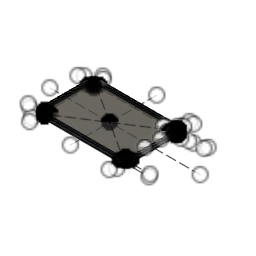
cover_bottom v1 (Autodesk Fusion 360 design; units mm, degrees)
Autodesk Fusion 360 part; units mm, degrees
note: some values were not read from the file. Set by a fixed rule: the direction of a hole.
sketch "Skizze1" plane through (0, 0, 0) normal (0, 0, 1) x (1, 0, 0)
  line L0 (85, -55) -> (-85, -55) construction
  line L1 (-85, -55) -> (-85, 55) construction
  line L2 (-85, 55) -> (85, 55) construction
  line L3 (85, 55) -> (85, -55) construction
  line L4 (85, -55) -> (-85, 55) construction
  line L5 (-85, -55) -> (85, 55) construction
  line L6 (83.8, -53.8) -> (-83.8, -53.8) construction
  line L7 (-83.8, -53.8) -> (-83.8, 53.8) construction
  line L8 (-83.8, 53.8) -> (83.8, 53.8) construction
  line L9 (83.8, 53.8) -> (83.8, -53.8) construction
  line L10 (83.8, -53.8) -> (-83.8, 53.8) construction
  line L11 (-83.8, -53.8) -> (83.8, 53.8) construction
  line L12 (60, 45) -> (112.6344, 45) construction
  line L13 (75, 65.4743) -> (75, 20.9271) construction
  arc A0 (85, 45) -> (75, 55) centre (75, 45) ccw
  line L14 (74, 76.2401) -> (74, -7.7296) construction
  line L15 (56.5373, 44) -> (104.4576, 44) construction
  arc A1 (83.8, 44) -> (74, 53.8) centre (74, 44) ccw
  line L16 (69, 40.8) -> (92.7084, 40.8) construction
  line L17 (70.8, 58.1175) -> (70.8, 37.2449) construction
  line L18 (-99.6173, 51.6) -> (133.2089, 51.6) construction
  line L19 (-98.318, -51.6) -> (125.4134, -51.6) construction
  line L20 (-81.6, 68.7546) -> (-81.6, -65.5882) construction
  line L21 (81.6, 76.2401) -> (81.6, -68.4466) construction
  line L22 (0, 88.5072) -> (0, -73.8187) construction
  line L23 (-112.3323, 0) -> (170, 0) construction
  arc A2 (-75, 55) -> (-85, 45) centre (-75, 45) ccw
  arc A3 (-74, 53.8) -> (-83.8, 44) centre (-74, 44) ccw
  arc A4 (75, -55) -> (85, -45) centre (75, -45) ccw
  arc A5 (74, -53.8) -> (83.8, -44) centre (74, -44) ccw
  arc A6 (-83.8, -44) -> (-74, -53.8) centre (-74, -44) ccw
  arc A7 (-85, -45) -> (-75, -55) centre (-75, -45) ccw
  line L24 (-85, 45) -> (-85, -45)
  line L25 (-83.8, -44) -> (-83.8, 44)
  line L26 (-75, 55) -> (75, 55)
  line L27 (74, 53.8) -> (-74, 53.8)
  line L28 (85, 45) -> (85, -45)
  line L29 (83.8, -44) -> (83.8, 44)
  line L30 (75, -55) -> (-75, -55)
  line L31 (-74, -53.8) -> (74, -53.8)
  line L32 (70.8, -51.6) -> (70.8, -40.8)
  line L33 (70.8, -40.8) -> (81.6, -40.8)
  line L34 (81.6, -40.8) -> (81.6, 40.8)
  line L35 (81.6, 40.8) -> (70.8, 40.8)
  line L36 (70.8, 40.8) -> (70.8, 51.6)
  line L37 (70.8, 51.6) -> (-70.8, 51.6)
  line L38 (-70.8, 40.8) -> (-71, 40.8)
  line L39 (-70.8, 51.6) -> (-70.8, 40.8)
  line L40 (-71, 40.8) -> (-81.6, 40.8)
  line L41 (-81.6, 40.8) -> (-81.6, -40.8)
  line L42 (-81.6, -40.8) -> (-70.8, -40.8)
  line L43 (-70.8, -40.8) -> (-70.8, -51.6)
  line L44 (-70.8, -51.6) -> (70.8, -51.6)
  line L45 (-105.874, 46.3) -> (130.8939, 46.3) construction
  line L46 (-106.5857, -46.3) -> (122.1159, -46.3) construction
  line L47 (76.3, 62.7556) -> (76.3, -77.2174) construction
  line L48 (-76.3, 64.1791) -> (-76.3, -73.896) construction
  circle A8 centre (76.3, 46.3) radius 4.5
  circle A9 centre (76.3, 46.3) radius 3
  circle A10 centre (76.3, -46.3) radius 4.5
  circle A11 centre (76.3, -46.3) radius 3
  circle A12 centre (-76.3, -46.3) radius 4.5
  circle A13 centre (-76.3, -46.3) radius 3
  circle A14 centre (-76.3, 46.3) radius 4.5
  circle A15 centre (-76.3, 46.3) radius 3
  line L49 (-68.8, 49.6) -> (68.8, 49.6)
  line L50 (68.8, 49.6) -> (68.8, 38.8)
  line L51 (68.8, 38.8) -> (79.6, 38.8)
  line L52 (79.6, 38.8) -> (79.6, -38.8)
  line L53 (79.6, -38.8) -> (68.8, -38.8)
  line L54 (68.8, -38.8) -> (68.8, -49.6)
  line L55 (68.8, -49.6) -> (-68.8, -49.6)
  line L56 (-68.8, -49.6) -> (-68.8, -38.8)
  line L57 (-68.8, -38.8) -> (-79.6, -38.8)
  line L58 (-79.6, -38.8) -> (-79.6, 38.8)
  line L59 (-79.6, 38.8) -> (-68.8, 38.8)
  line L60 (-68.8, 38.8) -> (-68.8, 49.6)
  point P0 (75, 45)
  point P1 (75, 55)
  point P2 (85, 45)
  point P3 (74, 44)
  point P4 (74, 53.8)
  point P5 (83.8, 44)
  point P6 (70.8, 51.6)
  point P7 (70.8, 40.8)
  point P8 (81.6, 40.8)
  point P9 (-81.6, 40.8)
  point P10 (-70.8, 51.6)
  point P11 (-70.8, 40.8)
  point P12 (81.6, -40.8)
  point P13 (70.8, -40.8)
  point P14 (70.8, -51.6)
  point P15 (-81.6, -40.8)
  point P16 (-70.8, -40.8)
  point P17 (-70.8, -51.6)
  point P18 (76.3, 46.3)
  point P19 (76.3, -46.3)
  point P20 (-76.3, -46.3)
  point P21 (-76.3, 46.3)
  dimension "d1" = 170
  dimension "d2" = 110
  dimension "d3" = 167.6
  dimension "d4" = 107.6
  dimension "d6" = 10
  dimension "d7" = 10
  dimension "d8" = 74
  dimension "d9" = 44
  dimension "d13" = 14.2
  dimension "d14" = 14.2
  dimension "d15" = 2.2
  dimension "d16" = 2.2
  dimension "d17" = 2.2
  dimension "d18" = 2.2
  dimension "d19" = 46.3
  dimension "d20" = 46.3
  dimension "d21" = 76.3
  dimension "d22" = 76.3
  dimension "d23" = 9
  dimension "d24" = 6
  dimension "d25" = 9
  dimension "d26" = 6
  dimension "d27" = 9
  dimension "d28" = 6
  dimension "d29" = 9
  dimension "d30" = 6
  dimension "d31" = 2
  dimension "d32" = 2
  dimension "d33" = 2
  dimension "d34" = 2
  dimension "d35" = 2
  dimension "d36" = 2
  dimension "d37" = 2
  dimension "d38" = 2
  dimension "d39" = 2
  dimension "d40" = 2
  dimension "d41" = 2
  dimension "d42" = 2
  constraint horizontal L0
  constraint perpendicular L0 L1
  constraint parallel L0 L2
  constraint parallel L1 L3
  constraint coincident L4 origin
  constraint coincident L5 origin
  constraint horizontal L6
  constraint perpendicular L6 L7
  constraint parallel L6 L8
  constraint parallel L7 L9
  constraint coincident L10 origin
  constraint coincident L11 origin
  constraint parallel L8 L12
  constraint perpendicular L2 L13
  constraint coincident L12 P0
  constraint coincident L13 P0
  constraint coincident L2 P1
  constraint coincident L13 P1
  constraint coincident L3 P2
  constraint coincident L12 P2
  constraint coincident P2 A0.start
  constraint coincident P1 A0.end
  constraint vertical L14
  constraint horizontal L15
  constraint coincident L15 P3
  constraint coincident L14 P3
  constraint coincident L8 P4
  constraint coincident L14 P4
  constraint coincident L15 P5
  constraint coincident L9 P5
  constraint coincident P5 A1.start
  constraint coincident P4 A1.end
  constraint parallel L15 L16
  constraint perpendicular L16 L17
  constraint perpendicular L1 L18
  constraint perpendicular L3 L19
  constraint perpendicular L0 L20
  constraint vertical L21
  constraint coincident L17 P6
  constraint coincident L18 P6
  constraint coincident L17 P7
  constraint coincident L16 P7
  constraint coincident L16 P8
  constraint coincident L21 P8
  constraint perpendicular L0 L22
  constraint horizontal L23
  constraint coincident origin L22
  constraint coincident origin L23
  constraint symmetric P2 L22 A2.end
  constraint symmetric P1 L22 A2.start
  constraint symmetric A0 L22 A2
  constraint symmetric P5 L22 A3.end
  constraint symmetric P4 L22 A3.start
  constraint symmetric A1 L22 A3
  constraint symmetric P6 L22 P10
  constraint symmetric P7 L22 P11
  constraint symmetric P8 L22 P9
  constraint symmetric P2 L23 A4.end
  constraint symmetric P1 L23 A4.start
  constraint symmetric A0 L23 A4
  constraint symmetric P5 L23 A5.end
  constraint symmetric P4 L23 A5.start
  constraint symmetric A1 L23 A5
  constraint symmetric P6 L23 P14
  constraint symmetric P7 L23 P13
  constraint symmetric P8 L23 P12
  constraint symmetric L23 P9 P15
  constraint symmetric L23 P10 P17
  constraint symmetric L23 P11 P16
  constraint symmetric L23 A2.end A7.start
  constraint symmetric L23 A2.start A7.end
  constraint symmetric L23 A2 A7
  constraint symmetric L23 A3.end A6.start
  constraint symmetric L23 A3.start A6.end
  constraint symmetric L23 A3 A6
  constraint tangent A7 L24
  constraint tangent A3 L25
  constraint tangent A0 L26
  constraint coincident P14 L32.start
  constraint coincident P13 L32.end
  constraint coincident P12 L33.end
  constraint coincident P8 L34.end
  constraint coincident P7 L35.end
  constraint coincident P6 L36.end
  constraint coincident P10 L37.end
  constraint coincident P11 L38.start
  constraint coincident P9 L40.end
  constraint perpendicular L20 L40
  constraint coincident P15 L41.end
  constraint coincident P16 L42.end
  constraint coincident P17 L43.end
  constraint horizontal L45
  constraint perpendicular L3 L46
  constraint perpendicular L44 L47
  constraint perpendicular L6 L48
  constraint coincident L47 P18
  constraint coincident L45 P18
  constraint coincident L47 P19
  constraint coincident L46 P19
  constraint coincident L48 P20
  constraint coincident L46 P20
  constraint coincident L48 P21
  constraint coincident L45 P21
  constraint coincident P18 A8.centre
  constraint concentric A8 A9
  constraint coincident P19 A10.centre
  constraint concentric A10 A11
  constraint coincident P20 A12.centre
  constraint coincident P21 A14.centre
  constraint concentric A14 A15
  constraint parallel L45 L49
  constraint perpendicular L45 L50
  constraint perpendicular L50 L51
  constraint perpendicular L33 L52
  constraint perpendicular L52 L53
  constraint perpendicular L46 L54
  constraint perpendicular L43 L55
  constraint perpendicular L55 L56
  constraint perpendicular L48 L57
  constraint perpendicular L55 L58
  constraint perpendicular L48 L59
  constraint perpendicular L49 L60
  measures "d1" distance of L1 L3
  measures "d2" distance of L0 L2
  measures "d3" distance of L7 L9
  measures "d4" distance of L6 L8
  measures "d6" distance of L2 L12
  measures "d7" distance of L3 L13
  measures "d8" distance of origin L14
  measures "d9" distance of origin L15
  measures "d13" distance of L2 L16
  measures "d14" distance of L3 L17
  measures "d15" distance of L9 L21
  measures "d16" distance of L6 L19
  measures "d17" distance of L7 L20
  measures "d18" distance of L8 L18
  measures "d19" distance of origin L45
  measures "d20" distance of L23 L46
  measures "d21" distance of L22 L47
  measures "d22" distance of L22 L48
  measures "d23" diameter of A8
  measures "d24" diameter of A9
  measures "d25" diameter of A10
  measures "d26" diameter of A11
  measures "d27" diameter of A12
  measures "d28" diameter of A13
  measures "d29" diameter of A14
  measures "d30" diameter of A15
  measures "d31" distance of L37 L49
  measures "d32" distance of L36 L50
  measures "d33" distance of L35 L51
  measures "d34" distance of L21 L52
  measures "d35" distance of L33 L53
  measures "d36" distance of L32 L54
  measures "d37" distance of L44 L55
  measures "d38" distance of L43 L56
  measures "d39" distance of L42 L57
  measures "d40" distance of L41 L58
  measures "d41" distance of L40 L59
  measures "d42" distance of L39 L60
extrude "Extrusion1" add sketch "Skizze1" along normal blind 2 contours A1 A3 A5 A6 L25 L27 L29 L31 | A8 | A9 | A10 | A11 | A12 | A13 | A14 | A15 | L49 L50 L51 L52 L53 L54 L55 L56 L57 L58 L59 L60 makes body 1 at (-22.9333, 12.9333, 0) makes body 2 at (-73.6328, 48.2148, 0)
extrude "Extrusion2" add sketch "Skizze1" along normal blind 5 separate body contours A8 | A9 | A10 | A11 | A12 | A13 | A14 | A15 makes body 3 at (-75.0812, -41.9682, 3.3333) makes body 4 at (77.5188, -41.9682, 3.3333) makes body 5 at (-75.0812, 50.6318, 3.3333) makes body 6 at (77.5188, 50.6318, 3.3333)
hole "Bohrung2" at (-76.3, 46.3, 0) at (-76.3, -46.3, 0) at (76.3, -46.3, 0) at (76.3, 46.3, 0) direction (0, 0, 1) diameter 3.5 depth 15 tip angle 180 bodies 2 3 4 5 6
extrude "Extrusion3" cut sketch "Skizze1" along normal blind 3 contours A9 | A11 | A13 | A15 bodies 2 3 4 5 6
extrude "Extrusion4" add sketch "Skizze1" along normal blind 5 contours A0 A2 A4 A7 L24 L26 L28 L30 | L32 L33 L34 L35 L36 L37 L38 L39 L40 L41 L42 L43 L44 bodies 1 2
